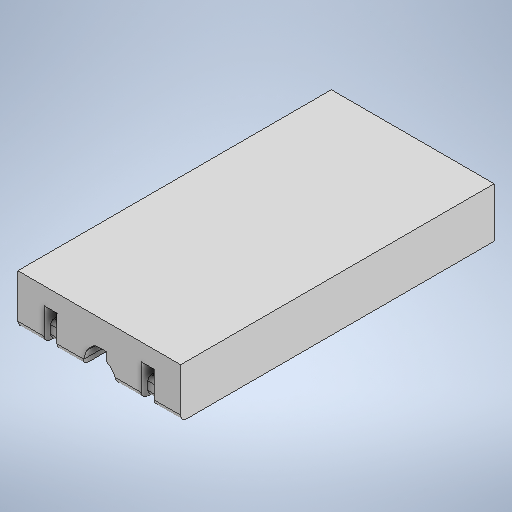
# Autodesk Inventor part: Laser_Pen_Housing_Top
Saved by Autodesk Inventor 2025 (Build 290162000, 162)
## iProperties
Created: 2024-05-23
Part Number: Laser_Pen_Housing_Top
Material: Generic
Document SubType Name: Modeling
Designer: mumin
Density: 1 g/cm^3
Appearance: Default
Author: mumin
Autodesk Inventor part; units mm, degrees
ref_plane "XZ Plane" through (0, 0, 0) normal (0, 1, 0) x (-1, 0, 0)
ref_plane "XY Plane" through (0, 0, 0) normal (0, 0, 1) x (1, 0, 0)
sketch "Sketch1" plane through (0, 0, 0) normal (0, 0, 1) x (1, 0, 0)
  line L0 (0, 0) -> (0, 44.0101) construction
  line L1 (-33.5, 0) -> (-6.975, 0)
  line L2 (6.975, 0) -> (33.5, 0)
  arc A0 (6.975, 0) -> (-6.975, 0) centre (0, 0) ccw
  line L3 (33.5, 0) -> (33.5, 20.5)
  line L4 (33.5, 20.5) -> (-33.5, 20.5)
  line L5 (-33.5, 20.5) -> (-33.5, 0)
  constraints: 12 end point, 2 horizontal, 2 point on circle, 1 centre point, 1 vertical
ref_plane "Work Plane1" through (20, 0, 0) normal (1, 0, 0) x (0, 1, 0)
extrude "Extrusion3" add sketch "Sketch1" along normal mid plane 129
sketch "Sketch4" plane through (20, 0, 0) normal (1, 0, 0) x (0, 1, 0)
  line L0 (0, 64.5) -> (0, -64.5) projected
  line L1 (2, 64.6) -> (10.1, 64.6)
  arc A0 (8, 56.9) -> (9.8375, 57.9834) centre (8, 59) ccw
  line L2 (8, 56.9) -> (4.9024, 56.9)
  arc A1 (6.2736, 58.9704) -> (4.9024, 56.9) centre (7, 57) ccw
  line L3 (6.9278, 59.9087) -> (6.9278, 60.4)
  line L4 (5.4278, 61.9) -> (2, 61.9)
  arc A2 (2, 61.9) -> (0.1051, 60.1387) centre (2, 60) ccw
  line L5 (0.1051, 60.1387) -> (0, 58.7036)
  line L6 (0, 62.6) -> (0, 58.7036)
  line L7 (0, -64.5) -> (0, 64.5) projected
  arc A3 (2, 64.6) -> (0, 62.6) centre (2, 62.6) ccw
  arc A4 (6.9278, 60.4) -> (5.4278, 61.9) centre (5.4278, 60.4) ccw
  line L8 (9.8375, 57.9834) -> (13.4982, 64.6)
  line L9 (13.4982, 64.6) -> (10.1, 64.6)
  arc A5 (6.2736, 58.9704) -> (6.9278, 59.9087) centre (5.9278, 59.9087) ccw
  point P0 (0, 0)
  point P1 (0, 64.6)
  point P2 (8, 64.6)
  point P3 (10.1, 62.5)
  point P4 (6.9278, 59.0988)
  point P5 (6.9278, 61.9)
  point P6 (0, 62.6)
  dimension "d33" = 2
  dimension "d34" = 1.5
  dimension "d35" = 1
  constraints: 16 end point, 13 point on circle, 8 tangent, 7 point on line, 6 centre point, 1 collinear
  measures "d33" radius of A3
  measures "d34" radius of A4
  measures "d35" radius of A5
extrude "Extrusion4" cut sketch "Sketch4" along normal mid plane 5.2
mirror "Mirror2" about plane through (0, 0, 0) normal (1, 0, 0) of "Extrusion4"
sketch "Sketch5" plane through (33.5, 0, 64.5) normal (1, 0, 0) x (0, 0, -1)
  line L0 (1.9, 0) -> (5.7964, 0) projected
  arc A0 (0, 2.5) -> (2.5, 0) centre (2.5, 2.5) ccw
  line L1 (2.5, 2.5) -> (2.5, 0) construction
  line L2 (2.5, 2.5) -> (5, 2.5) construction
  line L3 (2.5, 2.5) -> (0, 2.5) construction
  line L4 (0, 0) -> (0, 20.5) projected
  line L5 (0, 2.5) -> (0, 0)
  line L6 (0, 0) -> (129, 0) projected
  point P0 (64.5, 0)
  dimension "d36" = 90
  dimension "d37" = 90
  dimension "d38" = 2.5
  constraints: 8 end point, 2 point on circle, 2 point on line, 1 centre point, 1 collinear, 1 horizontal, 1 perpendicular
  measures "d36" angle of L1 L2
  measures "d37" angle of L3 L1
  measures "d38" distance of L1.start L3.end
extrude "Extrusion5" cut sketch "Sketch5" against normal through all
sketch "Sketch6" plane through (0, 0, 64.5) normal (0, 0, 1) x (1, 0, 0)
  arc A0 (6.5116, 2.5) -> (-6.5116, 2.5) centre (0, 0) ccw projected
  line L0 (0, 6.975) -> (2.875, 6.975) construction
  line L1 (2.875, 6.975) -> (2.875, 9.895) construction
  line L2 (-17.4, 0) -> (-6.975, 0) projected
  line L3 (2.875, 9.895) -> (2.875, 6.3549)
  spline S0 degree 6 poles (-6.5116, 2.5) (-6.5776, 2.3279) (-6.6388, 2.1522) (-6.6938, 1.976) (-6.7418, 1.8023) (-6.7828, 1.6341) (-6.8262, 1.4334) (-6.8346, 1.3932) (-6.8426, 1.3535) (-6.8502, 1.3144) (-6.8574, 1.2759) (-6.8768, 1.1683) (-6.8881, 1.1008) (-6.8982, 1.0356) (-6.9073, 0.9727) (-6.9153, 0.9122) (-6.9314, 0.7817) (-6.939, 0.7131) (-6.9453, 0.6483) (-6.9506, 0.5874) (-6.955, 0.5303) (-6.9696, 0.3178) (-6.9738, 0.1923) (-6.9749, 0.099) (-6.975, 0.0363) (-6.975, 0.0034) (-6.975, 0.0002) knots 0 0 0 0 0 0 0 0.246271 0.246271 0.246271 0.246271 0.246271 0.309061 0.309061 0.309061 0.309061 0.309061 0.424616 0.424616 0.424616 0.424616 0.424616 0.569008 0.569008 0.569008 0.569008 0.569008 1 1 1 1 1 1 1 projected
  line L4 (2.875, 9.895) -> (-0.5799, 9.895)
  line L5 (-2.875, 9.895) -> (-2.875, 8.895) construction
  arc A1 (-2.409, 9.2729) -> (-5.2406, 6.1296) centre (4.7239, 0) ccw
  arc A2 (-0.5799, 9.895) -> (-2.409, 9.2729) centre (-0.5799, 6.895) ccw
  line L6 (-6.5813, 2.3101) -> (-5.2406, 6.1296)
  point P0 (-1.5174, 9.895)
  dimension "d41" = 2.875
  dimension "d42" = 2.92
  dimension "d50" = 5.75
  dimension "d52" = 3
  constraints: 12 end point, 8 point on circle, 4 tangent, 3 point on line, 2 centre point, 2 horizontal, 1 perpendicular, 1 vertical, 3 other
  measures "d41" distance of L0.start L0.end
  measures "d42" distance of L0.end L1.end
  measures "d50" distance of L1.end L5.start
  measures "d52" radius of A2
sketch "Sketch7" plane through (0, 0, -64.5) normal (0, 0, -1) x (-1, 0, 0)
  arc A0 (6.975, 0) -> (-6.975, 0) centre (0, 0) ccw construction
  line L0 (0, 6.975) -> (-2.25, 6.975) construction
  line L1 (-2.25, 6.975) -> (-2.25, 10.675) construction
  arc A1 (8.1198, 7.2861) -> (-2.25, 10.675) centre (0, 0) ccw
  line L2 (0, 0) -> (8.1198, 7.2861) construction
  line L3 (0, 0) -> (-2.25, 10.675) construction
  line L4 (-2.25, 10.675) -> (-2.25, 6.6021)
  line L5 (8.1198, 7.2861) -> (5.1914, 4.6583)
  arc A2 (5.1914, 4.6583) -> (-2.25, 6.6021) centre (0, 0) ccw
  dimension "d45" = 2.25
  dimension "d46" = 3.7
  dimension "d47" = 60
  constraints: 12 end point, 7 point on circle, 2 centre point, 2 coincident, 2 point on line, 1 horizontal, 1 perpendicular, 1 tangent
  measures "d45" distance of L0.start L0.end
  measures "d46" distance of L0.end L1.end
  measures "d47" angle of L2 L3
extrude "Extrusion7" cut sketch "Sketch7" against normal blind 30
extrude "Extrusion8" cut sketch "Sketch6" against normal blind 56.46
body "Solid2"
